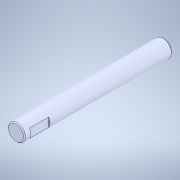
# Autodesk Inventor part: Motor Shaft
Saved by Autodesk Inventor 2022.2 (Build 262287030, 287C)
## iProperties
Created: 2016-08-15
Part Number: Motor Shaft
Material: SolidWorks DIN Materials|1.4000 (X6Cr13)
Document SubType Name: Modeling
Designer: Jochen
Density: 7.7 g/cm^3
Appearance: 202,209,238
Sending System: SolidWorks 2017
Last Author: Felix
Last Saved: 2019-07-15
Author: Jochen
Autodesk Inventor part; units mm, degrees
ref_plane "YZ Plane" through (0, 0, 0) normal (1, 0, 0) x (0, 1, 0)
ref_plane "XZ Plane" through (0, 0, 0) normal (0, 1, 0) x (-1, 0, 0)
ref_plane "XY Plane" through (0, 0, 0) normal (0, 0, 1) x (1, 0, 0)
sketch "Sketch1" plane through (0, 0, 0) normal (0, 0, 1) x (1, 0, 0)
  circle A0 centre (0, 0) radius 2
  dimension "d0" = 4
  constraints: 1 centre point, 1 coincident
  measures "d0" diameter of A0
extrude "Extrusion1" add sketch "Sketch1" along normal blind 34.9
chamfer "Chamfer1" distance 0.25 angle 45 2 edges at (-2, 0, 0) (-2, 0, 34.9)
sketch "Sketch3" plane through (0, 0, 0) normal (1, 0, 0) x (0, 1, 0)
  line L0 (2.5, 28.9) -> (-2.5, 28.9)
  line L1 (-2.5, 28.9) -> (-2.5, 33.4)
  line L2 (-2.5, 33.4) -> (2.5, 33.4)
  line L3 (2.5, 33.4) -> (2.5, 28.9)
  line L4 (-1.75, 34.9) -> (1.75, 34.9) projected
  line L5 (0, -6.9) -> (0, 41.4) construction
  line L6 (0, 0) -> (0, 1)
  line L7 (0, 1) -> (-1, 0)
  line L8 (-1, 0) -> (0, 0)
  line L9 (1.75, 0) -> (-1.75, 0) projected
  dimension "d6" = 1.5
  dimension "d7" = 4.5
  dimension "d8" = 5
  dimension "d13" = 1
  constraints: 14 end point, 2 parallel, 2 perpendicular, 2 point on line, 1 horizontal, 1 other
  measures "d6" distance between parallel lines of L4 L2
  measures "d7" distance of L0.end L1.end
  measures "d8" distance of L0.start L0.end
  measures "d13" distance of L7.end L6.start
extrude "Extrusion2" add sketch "Sketch3" along normal mid plane 10 separate body contours L0 L1 L2 L3
extrude "Extrusion3" cut sketch "Sketch3" along normal mid plane 3.4 contours L0 L1 L2 L3 bodies 2
combine bodies "Combine1" operation type subtract main body 1 bodies to subtract 2
revolve "Revolution1" cut sketch "Sketch3" angle 360 about axis through (0, 0, -10) along (0, 0, 1) bodies 1 contours L8 L7 L6
body "Solid1"
body "Solid2"
